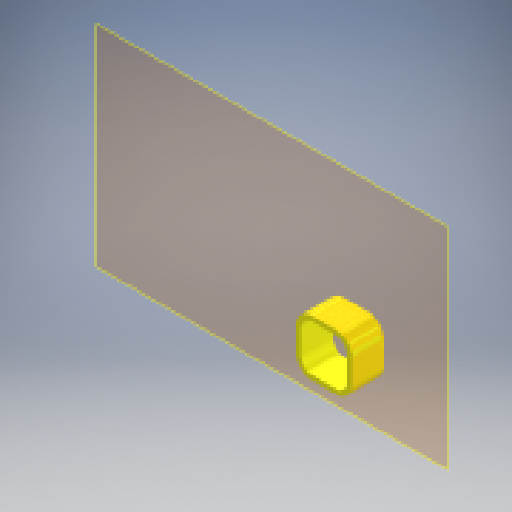
# Autodesk Inventor part: CE-8.2.2-01-004
Saved by Autodesk Inventor 2024 (Build 280153000, 153)
## iProperties
Created: 2024-03-07
Part Number: CE-8.2.2-01-004
Material: Generic
Document SubType Name: Modeling
Designer: Alex
Density: 1 g/cm^3
Appearance: Yellow
Author: Alex
Autodesk Inventor part; units mm, degrees
ref_plane "YZ Plane" through (0, 0, 0) normal (1, 0, 0) x (0, 1, 0)
ref_plane "XZ Plane" through (0, 0, 0) normal (0, 1, 0) x (-1, 0, 0)
ref_plane "XY Plane" through (0, 0, 0) normal (0, 0, 1) x (1, 0, 0)
ref_plane "Work Plane1" through (44.003, -30.6729, -33.7942) normal (0, 0, 1) x (1, 0, 0)
sketch "Sketch1" plane through (44.003, -30.6729, -33.7942) normal (0, 0, 1) x (1, 0, 0)
  line L0 (145, 55) -> (160, 55)
  arc A0 (145, 55) -> (135, 45) centre (145, 45) ccw
  line L1 (135, 30) -> (135, 45)
  arc A1 (135, 30) -> (145, 20) centre (145, 30) ccw
  line L2 (160, 20) -> (145, 20)
  arc A2 (160, 20) -> (170, 30) centre (160, 30) ccw
  line L3 (170, 45) -> (170, 30)
  arc A3 (170, 45) -> (160, 55) centre (160, 45) ccw
  point P0 (-44.003, 30.6729)
  constraints: 8 end point, 8 point on circle, 4 centre point, 2 horizontal, 2 vertical, 16 other
surface extrude "ExtrusionSrf1" sketch "Sketch1" along normal blind 20 shown yes curves A3 L0 A0 L1 A1 L2 A2 L3
thicken "Thicken1" operation new thickness 3 both sides no extend neighbours no toward (-0.7330519, 0.6801727, 0) faces at (211.3335, -7.4746, -20.4609) (214.003, 4.3271, -27.1276) (210.8047, 21.6576, -20.4609) (199.003, 24.3271, -27.1276) (181.6724, 21.1289, -20.4609) (179.003, 9.3271, -27.1276) (188.2557, -10.6449, -20.4609) (194.003, -10.6729, -27.1276)
body "Solid1"
body "Srf1"
